Autodesk Inventor part; units mm, degrees
(part 3 of 3)
  line L1573 (126.0856, -112.7887) -> (126.0856, -111.3282)
  line L1574 (126.0856, -111.3282) -> (126.6444, -111.3282)
  line L1575 (126.6444, -111.3282) -> (126.6444, -112.7887)
  line L1576 (127.9144, -112.7887) -> (127.3556, -112.7887)
  line L1577 (127.3556, -112.7887) -> (127.3556, -111.3282)
  line L1578 (127.3556, -111.3282) -> (127.9144, -111.3282)
  line L1579 (127.9144, -111.3282) -> (127.9144, -112.7887)
  line L1580 (129.1844, -112.7887) -> (128.6256, -112.7887)
  line L1581 (128.6256, -112.7887) -> (128.6256, -111.3282)
  line L1582 (128.6256, -111.3282) -> (129.1844, -111.3282)
  line L1583 (129.1844, -111.3282) -> (129.1844, -112.7887)
  line L1584 (134.2644, -112.7887) -> (133.7056, -112.7887)
  line L1585 (133.7056, -112.7887) -> (133.7056, -111.3282)
  line L1586 (133.7056, -111.3282) -> (134.2644, -111.3282)
  line L1587 (134.2644, -111.3282) -> (134.2644, -112.7887)
  line L1588 (132.9944, -112.7887) -> (132.4356, -112.7887)
  line L1589 (132.4356, -112.7887) -> (132.4356, -111.3282)
  line L1590 (132.4356, -111.3282) -> (132.9944, -111.3282)
  line L1591 (132.9944, -111.3282) -> (132.9944, -112.7887)
  line L1592 (131.7244, -112.7887) -> (131.1656, -112.7887)
  line L1593 (131.1656, -112.7887) -> (131.1656, -111.3282)
  line L1594 (131.1656, -111.3282) -> (131.7244, -111.3282)
  line L1595 (131.7244, -111.3282) -> (131.7244, -112.7887)
  line L1596 (130.4544, -112.7887) -> (129.8956, -112.7887)
  line L1597 (129.8956, -112.7887) -> (129.8956, -111.3282)
  line L1598 (129.8956, -111.3282) -> (130.4544, -111.3282)
  line L1599 (130.4544, -111.3282) -> (130.4544, -112.7887)
  point P0 (0, 0)
  constraints: 3200 end point
extrude "Extrusion2" add sketch "Sketch2" along normal blind 0.01
body "Solid1"
